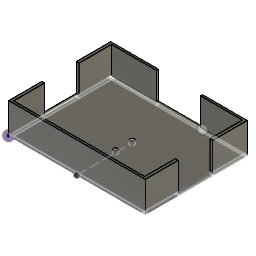
top (Autodesk Fusion 360 design; units mm, degrees)
part number: 2026-01-02-18-49-30-717
Autodesk Fusion 360 part; units mm, degrees
sketch "Szkic1" plane through (0, 0, 0) normal (0, 0, 1) x (1, 0, 0)
  line L0 (0, 0) -> (99, 0)
  line L1 (99, 0) -> (99, 74)
  line L2 (99, 74) -> (0, 74)
  line L3 (0, 74) -> (0, 0)
  line L4 (0, 74) -> (2, 74)
  line L5 (2, 74) -> (2, 0)
  line L6 (0, 74) -> (0, 72.5)
  line L7 (0, 72.5) -> (99, 72.5)
  line L8 (0, 0) -> (0, 1.5)
  line L9 (0, 1.5) -> (99, 1.5)
  line L10 (99, 0) -> (97, 0)
  line L11 (97, 0) -> (97, 74)
  line L12 (0, 74) -> (34.5, 74)
  line L13 (34.5, 74) -> (34.5, 72.5)
  line L14 (66.5, 74) -> (66.5, 72.5)
  line L15 (0, 74) -> (0, 49)
  line L16 (0, 49) -> (2, 49)
  line L17 (0, 49) -> (0, 24)
  line L18 (0, 24) -> (2, 24)
  line L19 (99, 74) -> (99, 49)
  line L20 (99, 49) -> (97, 49)
  line L21 (99, 49) -> (99, 24)
  line L22 (99, 24) -> (97, 24)
  line L23 (49.5, 0) -> (49.5, 28) construction
  line L24 (49.5, 28) -> (49.5, 40) construction
  circle A0 centre (49.5, 40) radius 1.5
  circle A1 centre (49.5, 28) radius 1.5
  point P0 (49.5, 0)
  dimension "d1" = 99
  dimension "d2" = 74
  dimension "d3" = 2
  dimension "d5" = 2
  dimension "d6" = 34.5
  dimension "d7" = 32
  dimension "d8" = 25
  dimension "d9" = 25
  dimension "d10" = 25
  dimension "d11" = 25
  dimension "d18" = 3
  dimension "d19" = 3
  dimension "d22" = 28
  dimension "d23" = 12
  dimension "d26" = 1.5
  dimension "d27" = 1.5
  constraint horizontal L0
  constraint vertical L1
  constraint horizontal L2
  constraint vertical L3
  constraint coincident L0.start L3.end
  constraint horizontal L4
  constraint coincident L0 L5.end
  constraint perpendicular L0 L5
  constraint perpendicular L2 L6
  constraint coincident L1 L7.end
  constraint perpendicular L1 L7
  constraint coincident L3 L8.end
  constraint coincident L1 L9.end
  constraint perpendicular L1 L9
  constraint horizontal L10
  constraint coincident L2 L11.end
  constraint perpendicular L7 L11
  constraint perpendicular L5 L12
  constraint coincident L7 L13.end
  constraint perpendicular L7 L13
  constraint coincident L7 L14.end
  constraint perpendicular L7 L14
  constraint perpendicular L2 L15
  constraint coincident L5 L16.end
  constraint perpendicular L5 L16
  constraint perpendicular L16 L17
  constraint coincident L5 L18.end
  constraint perpendicular L5 L18
  constraint perpendicular L7 L19
  constraint coincident L11 L20.end
  constraint perpendicular L11 L20
  constraint perpendicular L20 L21
  constraint coincident L11 L22.end
  constraint perpendicular L11 L22
  constraint midpoint L0 P0
  constraint coincident P0 L23.start
  constraint perpendicular L9 L23
  constraint parallel L23 L24
  constraint coincident L24.end A0.centre
  constraint coincident L23.end L24.start
  measures "d1" distance of L0.start L0.end
  measures "d2" distance of L0.start L2.end
  measures "d3" distance of L2.end L4.end
  measures "d5" distance of L0.end L10.end
  measures "d6" distance of L2.end L12.end
  measures "d7" distance of L12.end L14.start
  measures "d8" distance of L2.end L15.end
  measures "d9" distance of L15.end L17.end
  measures "d10" distance of L1.end L19.end
  measures "d11" distance of L19.end L21.end
  measures "d18" diameter of A0
  measures "d19" diameter of A1
  measures "d22" distance of L0 L23.end
  measures "d23" distance of L24.end L23.end
  measures "d26" distance of L0 L9
  measures "d27" distance of L2 L7
extrude "Wyciągnięcie proste1" add sketch "Szkic1" along normal blind 22 contours L0 L3 L5 L8 L9 | L0 L5 L9 L11 | L3 L5 L9 L18 | L0 L1 L9 L10 L11 | L1 L9 L11 L22 | L3 L5 L7 L15 L16 | L2 L3 L4 L5 L6 L7 L12 L15 | L1 L7 L11 L19 L20 | L2 L5 L7 L12 L13 | L1 L2 L7 L11 L19 | L2 L7 L11 L14 makes body 1 at (33, 0, 7.3333) makes body 2 at (88.1667, 74, 14.6667) makes body 3 at (23, 74, 7.3333)
extrude "Wyciągnięcie proste2" add sketch "Szkic1" along normal blind 1 separate body contours L5 L7 L9 L11 | L3 L5 L16 L17 L18 | L1 L11 L20 L21 L22 | L2 L7 L13 L14 | A0 | A1 makes body 4
combine "Kombinacja1" operation add target body 4 tool bodies 3 1 2
extrude "Wyciągnięcie proste3" cut sketch "Szkic1" along normal blind 6 contours A0 | A1 bodies 4
extrude "Wyciągnięcie proste4" add 1 faces at (49.4799, 9.8337, 1) along direction (0, 0, 1) blind 1 on bodies 4 bodies 4
named bodies: "Bryła1"
